Autodesk Fusion 360 part; units mm, degrees
note: some values were not read from the file. Set by a fixed rule: which sketch regions a step uses.
(part 3 of 7)
  spline S11 degree 5 poles (5.9883, 0.3741) (5.9868, 0.3751) (5.9838, 0.377) (5.9792, 0.3799) (5.9731, 0.3838) (5.9655, 0.3886) (5.9579, 0.3934) (5.9503, 0.3981) (5.9427, 0.4028) (5.9352, 0.4075) (5.9276, 0.4121) (5.92, 0.4167) (5.9125, 0.4213) (5.905, 0.4259) (5.8974, 0.4304) (5.8899, 0.4349) (5.8824, 0.4393) (5.8749, 0.4437) (5.8674, 0.4481) (5.8599, 0.4525) (5.8524, 0.4568) (5.845, 0.4611) (5.8375, 0.4654) (5.8301, 0.4696) (5.8226, 0.4738) (5.8152, 0.478) (5.8078, 0.4821) (5.8004, 0.4862) (5.793, 0.4903) (5.7856, 0.4943) (5.7782, 0.4984) (5.7709, 0.5023) (5.7635, 0.5063) (5.7562, 0.5102) (5.7489, 0.5141) (5.7416, 0.518) (5.7343, 0.5218) (5.727, 0.5256) (5.7197, 0.5293) (5.7124, 0.5331) (5.7052, 0.5368) (5.6979, 0.5405) (5.6907, 0.5441) (5.6835, 0.5477) (5.6763, 0.5513) (5.6691, 0.5548) (5.662, 0.5584) (5.6548, 0.5618) (5.6477, 0.5653) (5.6405, 0.5687) (5.6334, 0.5721) (5.6263, 0.5755) (5.6192, 0.5788) (5.6122, 0.5821) (5.6051, 0.5854) (5.5981, 0.5887) (5.5911, 0.5919) (5.584, 0.5951) (5.5771, 0.5982) (5.5701, 0.6013) (5.5631, 0.6044) (5.5562, 0.6075) (5.5492, 0.6105) (5.5423, 0.6136) (5.5354, 0.6165) (5.5286, 0.6195) (5.5217, 0.6224) (5.5149, 0.6253) (5.508, 0.6281) (5.5012, 0.631) (5.4945, 0.6338) (5.4877, 0.6366) (5.4809, 0.6393) (5.4742, 0.642) (5.4675, 0.6447) (5.4608, 0.6473) (5.4541, 0.65) (5.4475, 0.6526) (5.4408, 0.6551) (5.4342, 0.6577) (5.4276, 0.6602) (5.421, 0.6627) (5.4145, 0.6651) (5.4079, 0.6676) (5.4014, 0.67) (5.3949, 0.6723) (5.3884, 0.6747) (5.382, 0.677) (5.3756, 0.6793) (5.3691, 0.6815) (5.3628, 0.6838) (5.3564, 0.686) (5.35, 0.6882) (5.3437, 0.6903) (5.3374, 0.6924) (5.3311, 0.6945) (5.3249, 0.6966) (5.3186, 0.6986) (5.3124, 0.7006) (5.3063, 0.7026) (5.3001, 0.7046) (5.294, 0.7065) (5.2878, 0.7084) (5.2817, 0.7103) (5.2757, 0.7122) (5.2696, 0.714) (5.2636, 0.7158) (5.2576, 0.7176) (5.2517, 0.7193) (5.2457, 0.721) (5.2398, 0.7227) (5.2339, 0.7244) (5.2281, 0.726) (5.2222, 0.7277) (5.2164, 0.7293) (5.2106, 0.7308) (5.2049, 0.7324) (5.1991, 0.7339) (5.1934, 0.7354) (5.1878, 0.7368) (5.1821, 0.7383) (5.1765, 0.7397) (5.1709, 0.7411) (5.1653, 0.7425) (5.1598, 0.7438) (5.1543, 0.7451) (5.1488, 0.7464) (5.1434, 0.7477) (5.1379, 0.749) (5.1326, 0.7502) (5.1272, 0.7514) (5.1219, 0.7526) (5.1166, 0.7537) (5.1113, 0.7549) (5.1061, 0.756) (5.1009, 0.7571) (5.0957, 0.7581) (5.0905, 0.7592) (5.0854, 0.7602) (5.0803, 0.7612) (5.0753, 0.7622) (5.0703, 0.7631) (5.0653, 0.7641) (5.0604, 0.765) (5.0554, 0.7659) (5.0506, 0.7667) (5.0457, 0.7676) (5.0409, 0.7684) (5.0361, 0.7692) (5.0314, 0.77) (5.0266, 0.7708) (5.022, 0.7715) (5.0173, 0.7722) (5.0127, 0.7729) (5.0081, 0.7736) (5.0036, 0.7743) (4.9991, 0.7749) (4.9946, 0.7755) (4.9902, 0.7762) (4.9858, 0.7767) (4.9815, 0.7773) (4.9771, 0.7779) (4.9729, 0.7784) (4.9686, 0.7789) (4.9644, 0.7794) (4.9602, 0.7799) (4.9561, 0.7803) (4.952, 0.7808) (4.948, 0.7812) (4.944, 0.7816) (4.94, 0.782) (4.9361, 0.7824) (4.9322, 0.7828) (4.9283, 0.7831) (4.9245, 0.7834) (4.9207, 0.7838) (4.917, 0.784) (4.9133, 0.7843) (4.9097, 0.7846) (4.9061, 0.7849) (4.9025, 0.7851) (4.899, 0.7853) (4.8955, 0.7855) (4.8921, 0.7857) (4.8887, 0.7859) (4.8853, 0.7861) (4.882, 0.7862) (4.8788, 0.7864) (4.8756, 0.7865) (4.8724, 0.7866) (4.8693, 0.7867) (4.8662, 0.7868) (4.8632, 0.7869) (4.8602, 0.787) (4.8572, 0.7871) (4.8543, 0.7871) (4.8515, 0.7872) (4.8487, 0.7872) (4.846, 0.7872) (4.8433, 0.7872) (4.8406, 0.7872) (4.838, 0.7872) (4.8354, 0.7872) (4.8329, 0.7872) (4.8305, 0.7872) (4.8281, 0.7871) (4.8257, 0.7871) (4.8234, 0.787) (4.8211, 0.787) (4.8189, 0.7869) (4.8168, 0.7868) (4.8147, 0.7868) (4.8126, 0.7867) (4.8106, 0.7866) (4.8087, 0.7865) (4.8068, 0.7864) (4.805, 0.7863) (4.8032, 0.7862) (4.8015, 0.7861) (4.7998, 0.786) (4.7982, 0.7859) (4.7966, 0.7858) (4.7951, 0.7857) (4.7937, 0.7856) (4.7923, 0.7854) (4.7909, 0.7853) (4.7896, 0.7852) (4.7884, 0.7851) (4.7873, 0.785) (4.7862, 0.7849) (4.7851, 0.7848) (4.7841, 0.7847) (4.7832, 0.7846) (4.7824, 0.7845) (4.7816, 0.7844) (4.7808, 0.7843) (4.7801, 0.7842) (4.7795, 0.7841) (4.779, 0.7841) (4.7785, 0.784) (4.778, 0.7839) (4.7778, 0.7839) (4.7776, 0.7839) (4.7775, 0.7838) (4.7774, 0.7838) knots -1 -1 -1 -1 -1 -1 -0.99583333 -0.99166667 -0.9875 -0.98333333 -0.97916667 -0.975 -0.97083333 -0.96666667 -0.9625 -0.95833333 -0.95416667 -0.95 -0.94583333 -0.94166667 -0.9375 -0.93333333 -0.92916667 -0.925 -0.92083333 -0.91666667 -0.9125 -0.90833333 -0.90416667 -0.9 -0.89583333 -0.89166667 -0.8875 -0.88333333 -0.87916667 -0.875 -0.87083333 -0.86666667 -0.8625 -0.85833333 -0.85416667 -0.85 -0.84583333 -0.84166667 -0.8375 -0.83333333 -0.82916667 -0.825 -0.82083333 -0.81666667 -0.8125 -0.80833333 -0.80416667 -0.8 -0.79583333 -0.79166667 -0.7875 -0.78333333 -0.77916667 -0.775 -0.77083333 -0.76666667 -0.7625 -0.75833333 -0.75416667 -0.75 -0.74583333 -0.74166667 -0.7375 -0.73333333 -0.72916667 -0.725 -0.72083333 -0.71666667 -0.7125 -0.70833333 -0.70416667 -0.7 -0.69583333 -0.69166667 -0.6875 -0.68333333 -0.67916667 -0.675 -0.67083333 -0.66666667 -0.6625 -0.65833333 -0.65416667 -0.65 -0.64583333 -0.64166667 -0.6375 -0.63333333 -0.62916667 -0.625 -0.62083333 -0.61666667 -0.6125 -0.60833333 -0.60416667 -0.6 -0.59583333 -0.59166667 -0.5875 -0.58333333 -0.57916667 -0.575 -0.57083333 -0.56666667 -0.5625 -0.55833333 -0.55416667 -0.55 -0.54583333 -0.54166667 -0.5375 -0.53333333 -0.52916667 -0.525 -0.52083333 -0.51666667 -0.5125 -0.50833333 -0.50416667 -0.5 -0.49583333 -0.49166667 -0.4875 -0.48333333 -0.47916667 -0.475 -0.47083333 -0.46666667 -0.4625 -0.45833333 -0.45416667 -0.45 -0.44583333 -0.44166667 -0.4375 -0.43333333 -0.42916667 -0.425 -0.42083333 -0.41666667 -0.4125 -0.40833333 -0.40416667 -0.4 -0.39583333 -0.39166667 -0.3875 -0.38333333 -0.37916667 -0.375 -0.37083333 -0.36666667 -0.3625 -0.35833333 -0.35416667 -0.35 -0.34583333 -0.34166667 -0.3375 -0.33333333 -0.32916667 -0.325 -0.32083333 -0.31666667 -0.3125 -0.30833333 -0.30416667 -0.3 -0.29583333 -0.29166667 -0.2875 -0.28333333 -0.27916667 -0.275 -0.27083333 -0.26666667 -0.2625 -0.25833333 -0.25416667 -0.25 -0.24583333 -0.24166667 -0.2375 -0.23333333 -0.22916667 -0.225 -0.22083333 -0.21666667 -0.2125 -0.20833333 -0.20416667 -0.2 -0.19583333 -0.19166667 -0.1875 -0.18333333 -0.17916667 -0.175 -0.17083333 -0.16666667 -0.1625 -0.15833333 -0.15416667 -0.15 -0.14583333 -0.14166667 -0.1375 -0.13333333 -0.12916667 -0.125 -0.12083333 -0.11666667 -0.1125 -0.10833333 -0.10416667 -0.1 -0.09583333 -0.09166667 -0.0875 -0.08333333 -0.07916667 -0.075 -0.07083333 -0.06666667 -0.0625 -0.05833333 -0.05416667 -0.05 -0.04583333 -0.04166667 -0.0375 -0.03333333 -0.02916667 -0.025 -0.02083333 -0.01666667 -0.0125 -0.00833333 -0.00416667 0 0 0 0 0 0
  line L22 (4.7774, 0.7838) -> (4.7769, 0.7838)
  line L23 (4.7769, 0.7838) -> (3.7005, 0.6072)
  arc A12 (3.7005, 0.6072) -> (3.3507, 1.6839) centre (0, 0) ccw
  line L24 (3.3507, 1.6839) -> (4.3252, 2.1737)
  line L25 (4.3252, 2.1737) -> (4.3257, 2.1739)
  spline S12 degree 5 poles (4.3257, 2.1739) (4.3258, 2.174) (4.3259, 2.174) (4.326, 2.1741) (4.3263, 2.1742) (4.3267, 2.1745) (4.3271, 2.1747) (4.3276, 2.175) (4.3282, 2.1753) (4.3288, 2.1756) (4.3294, 2.1759) (4.3301, 2.1763) (4.3309, 2.1768) (4.3317, 2.1772) (4.3325, 2.1777) (4.3334, 2.1782) (4.3344, 2.1788) (4.3354, 2.1794) (4.3364, 2.18) (4.3375, 2.1807) (4.3387, 2.1814) (4.3399, 2.1821) (4.3411, 2.1829) (4.3424, 2.1837) (4.3437, 2.1845) (4.3451, 2.1854) (4.3465, 2.1863) (4.348, 2.1872) (4.3495, 2.1881) (4.351, 2.1891) (4.3526, 2.1902) (4.3542, 2.1913) (4.3559, 2.1924) (4.3576, 2.1935) (4.3593, 2.1947) (4.3611, 2.1959) (4.363, 2.1971) (4.3648, 2.1984) (4.3667, 2.1997) (4.3686, 2.2011) (4.3706, 2.2025) (4.3726, 2.2039) (4.3747, 2.2053) (4.3767, 2.2068) (4.3788, 2.2084) (4.381, 2.2099) (4.3832, 2.2115) (4.3854, 2.2132) (4.3876, 2.2148) (4.3899, 2.2165) (4.3922, 2.2183) (4.3946, 2.22) (4.3969, 2.2219) (4.3993, 2.2237) (4.4018, 2.2256) (4.4042, 2.2275) (4.4067, 2.2295) (4.4092, 2.2315) (4.4118, 2.2335) (4.4144, 2.2356) (4.417, 2.2377) (4.4196, 2.2398) (4.4223, 2.242) (4.425, 2.2442) (4.4277, 2.2465) (4.4304, 2.2488) (4.4332, 2.2511) (4.436, 2.2534) (4.4388, 2.2558) (4.4416, 2.2583) (4.4445, 2.2607) (4.4474, 2.2632) (4.4503, 2.2658) (4.4532, 2.2684) (4.4562, 2.271) (4.4592, 2.2736) (4.4622, 2.2763) (4.4652, 2.279) (4.4683, 2.2818) (4.4713, 2.2846) (4.4744, 2.2874) (4.4775, 2.2903) (4.4807, 2.2932) (4.4838, 2.2962) (4.487, 2.2992) (4.4902, 2.3022) (4.4934, 2.3052) (4.4966, 2.3083) (4.4998, 2.3115) (4.5031, 2.3146) (4.5064, 2.3178) (4.5097, 2.3211) (4.513, 2.3244) (4.5163, 2.3277) (4.5197, 2.331) (4.523, 2.3344) (4.5264, 2.3378) (4.5298, 2.3413) (4.5332, 2.3448) (4.5367, 2.3483) (4.5401, 2.3519) (4.5435, 2.3555) (4.547, 2.3592) (4.5505, 2.3629) (4.554, 2.3666) (4.5575, 2.3703) (4.561, 2.3741) (4.5646, 2.378) (4.5681, 2.3818) (4.5717, 2.3857) (4.5752, 2.3897) (4.5788, 2.3937) (4.5824, 2.3977) (4.586, 2.4017) (4.5896, 2.4058) (4.5933, 2.4099) (4.5969, 2.4141) (4.6006, 2.4183) (4.6042, 2.4225) (4.6079, 2.4268) (4.6116, 2.4311) (4.6153, 2.4354) (4.619, 2.4398) (4.6227, 2.4442) (4.6264, 2.4487) (4.6301, 2.4532) (4.6338, 2.4577) (4.6376, 2.4623) (4.6413, 2.4668) (4.645, 2.4715) (4.6488, 2.4761) (4.6526, 2.4809) (4.6563, 2.4856) (4.6601, 2.4904) (4.6639, 2.4952) (4.6677, 2.5) (4.6715, 2.5049) (4.6753, 2.5098) (4.6791, 2.5148) (4.6829, 2.5198) (4.6867, 2.5248) (4.6905, 2.5299) (4.6944, 2.535) (4.6982, 2.5401) (4.702, 2.5453) (4.7058, 2.5505) (4.7097, 2.5557) (4.7135, 2.561) (4.7174, 2.5663) (4.7212, 2.5717) (4.7251, 2.5771) (4.7289, 2.5825) (4.7328, 2.5879) (4.7366, 2.5934) (4.7405, 2.599) (4.7443, 2.6045) (4.7482, 2.6101) (4.7521, 2.6158) (4.7559, 2.6214) (4.7598, 2.6271) (4.7636, 2.6329) (4.7675, 2.6386) (4.7714, 2.6444) (4.7752, 2.6503) (4.7791, 2.6562) (4.7829, 2.6621) (4.7868, 2.668) (4.7907, 2.674) (4.7945, 2.68) (4.7984, 2.6861) (4.8022, 2.6921) (4.8061, 2.6983) (4.8099, 2.7044) (4.8138, 2.7106) (4.8176, 2.7168) (4.8215, 2.7231) (4.8253, 2.7294) (4.8292, 2.7357) (4.833, 2.7421) (4.8368, 2.7484) (4.8407, 2.7549) (4.8445, 2.7613) (4.8483, 2.7678) (4.8521, 2.7744) (4.8559, 2.7809) (4.8597, 2.7875) (4.8636, 2.7941) (4.8674, 2.8008) (4.8712, 2.8075) (4.8749, 2.8142) (4.8787, 2.821) (4.8825, 2.8278) (4.8863, 2.8346) (4.8901, 2.8415) (4.8938, 2.8484) (4.8976, 2.8553) (4.9013, 2.8623) (4.9051, 2.8693) (4.9088, 2.8763) (4.9125, 2.8834) (4.9163, 2.8905) (4.92, 2.8976) (4.9237, 2.9047) (4.9274, 2.9119) (4.9311, 2.9192) (4.9348, 2.9264) (4.9385, 2.9337) (4.9421, 2.941) (4.9458, 2.9484) (4.9495, 2.9558) (4.9531, 2.9632) (4.9568, 2.9706) (4.9604, 2.9781) (4.964, 2.9856) (4.9676, 2.9932) (4.9712, 3.0008) (4.9748, 3.0084) (4.9784, 3.016) (4.982, 3.0237) (4.9855, 3.0314) (4.9891, 3.0391) (4.9927, 3.0469) (4.9962, 3.0547) (4.9997, 3.0625) (5.0032, 3.0704) (5.0067, 3.0783) (5.0102, 3.0862) (5.0137, 3.0942) (5.0172, 3.1022) (5.0206, 3.1102) (5.0241, 3.1182) (5.0275, 3.1263) (5.031, 3.1344) (5.0344, 3.1426) (5.0378, 3.1507) (5.0412, 3.1589) (5.0445, 3.1672) (5.0479, 3.1754) (5.0513, 3.1837) (5.0546, 3.192) (5.0579, 3.2004) (5.0606, 3.2071) (5.0626, 3.2121) (5.0639, 3.2155) (5.0645, 3.2172) knots 0 0 0 0 0 0 0.00416667 0.00833333 0.0125 0.01666667 0.02083333 0.025 0.02916667 0.03333333 0.0375 0.04166667 0.04583333 0.05 0.05416667 0.05833333 0.0625 0.06666667 0.07083333 0.075 0.07916667 0.08333333 0.0875 0.09166667 0.09583333 0.1 0.10416667 0.10833333 0.1125 0.11666667 0.12083333 0.125 0.12916667 0.13333333 0.1375 0.14166667 0.14583333 0.15 0.15416667 0.15833333 0.1625 0.16666667 0.17083333 0.175 0.17916667 0.18333333 0.1875 0.19166667 0.19583333 0.2 0.20416667 0.20833333 0.2125 0.21666667 0.22083333 0.225 0.22916667 0.23333333 0.2375 0.24166667 0.24583333 0.25 0.25416667 0.25833333 0.2625 0.26666667 0.27083333 0.275 0.27916667 0.28333333 0.2875 0.29166667 0.29583333 0.3 0.30416667 0.30833333 0.3125 0.31666667 0.32083333 0.325 0.32916667 0.33333333 0.3375 0.34166667 0.34583333 0.35 0.35416667 0.35833333 0.3625 0.36666667 0.37083333 0.375 0.37916667 0.38333333 0.3875 0.39166667 0.39583333 0.4 0.40416667 0.40833333 0.4125 0.41666667 0.42083333 0.425 0.42916667 0.43333333 0.4375 0.44166667 0.44583333 0.45 0.45416667 0.45833333 0.4625 0.46666667 0.47083333 0.475 0.47916667 0.48333333 0.4875 0.49166667 0.49583333 0.5 0.50416667 0.50833333 0.5125 0.51666667 0.52083333 0.525 0.52916667 0.53333333 0.5375 0.54166667 0.54583333 0.55 0.55416667 0.55833333 0.5625 0.56666667 0.57083333 0.575 0.57916667 0.58333333 0.5875 0.59166667 0.59583333 0.6 0.60416667 0.60833333 0.6125 0.61666667 0.62083333 0.625 0.62916667 0.63333333 0.6375 0.64166667 0.64583333 0.65 0.65416667 0.65833333 0.6625 0.66666667 0.67083333 0.675 0.67916667 0.68333333 0.6875 0.69166667 0.69583333 0.7 0.70416667 0.70833333 0.7125 0.71666667 0.72083333 0.725 0.72916667 0.73333333 0.7375 0.74166667 0.74583333 0.75 0.75416667 0.75833333 0.7625 0.76666667 0.77083333 0.775 0.77916667 0.78333333 0.7875 0.79166667 0.79583333 0.8 0.80416667 0.80833333 0.8125 0.81666667 0.82083333 0.825 0.82916667 0.83333333 0.8375 0.84166667 0.84583333 0.85 0.85416667 0.85833333 0.8625 0.86666667 0.87083333 0.875 0.87916667 0.88333333 0.8875 0.89166667 0.89583333 0.9 0.90416667 0.90833333 0.9125 0.91666667 0.92083333 0.925 0.92916667 0.93333333 0.9375 0.94166667 0.94583333 0.95 0.95416667 0.95833333 0.9625 0.96666667 0.97083333 0.975 0.97916667 0.98333333 0.9875 0.99166667 0.99583333 1 1 1 1 1 1
  arc A13 (5.0645, 3.2172) -> (4.6248, 3.8225) centre (0, 0) ccw
  spline S13 degree 5 poles (4.6248, 3.8225) (4.623, 3.8224) (4.6194, 3.8222) (4.6139, 3.8218) (4.6067, 3.8214) (4.5978, 3.8208) (4.5888, 3.8202) (4.5799, 3.8196) (4.571, 3.8189) (4.5621, 3.8183) (4.5533, 3.8176) (4.5445, 3.8169) (4.5357, 3.8161) (4.5269, 3.8154) (4.5181, 3.8146) (4.5094, 3.8138) (4.5007, 3.813) (4.4921, 3.8122) (4.4834, 3.8113) (4.4748, 3.8104) (4.4662, 3.8095) (4.4576, 3.8086) (4.4491, 3.8077) (4.4406, 3.8067) (4.4321, 3.8058) (4.4236, 3.8048) (4.4152, 3.8038) (4.4068, 3.8027) (4.3984, 3.8017) (4.3901, 3.8006) (4.3818, 3.7995) (4.3735, 3.7984) (4.3652, 3.7973) (4.357, 3.7962) (4.3488, 3.795) (4.3406, 3.7938) (4.3324, 3.7926) (4.3243, 3.7914) (4.3162, 3.7902) (4.3081, 3.789) (4.3001, 3.7877) (4.2921, 3.7864) (4.2841, 3.7851) (4.2761, 3.7838) (4.2682, 3.7825) (4.2603, 3.7811) (4.2524, 3.7797) (4.2446, 3.7783) (4.2368, 3.7769) (4.229, 3.7755) (4.2212, 3.7741) (4.2135, 3.7727) (4.2058, 3.7712) (4.1982, 3.7697) (4.1905, 3.7682) (4.1829, 3.7667) (4.1754, 3.7652) (4.1678, 3.7636) (4.1603, 3.7621) (4.1528, 3.7605) (4.1454, 3.7589) (4.138, 3.7573) (4.1306, 3.7557) (4.1232, 3.7541) (4.1159, 3.7524) (4.1086, 3.7508) (4.1013, 3.7491) (4.0941, 3.7474) (4.0869, 3.7457) (4.0797, 3.744) (4.0726, 3.7423) (4.0655, 3.7406) (4.0584, 3.7388) (4.0514, 3.7371) (4.0444, 3.7353) (4.0374, 3.7335) (4.0304, 3.7317) (4.0235, 3.7299) (4.0166, 3.7281) (4.0098, 3.7262) (4.003, 3.7244) (3.9962, 3.7225) (3.9894, 3.7207) (3.9827, 3.7188) (3.976, 3.7169) (3.9694, 3.715) (3.9628, 3.7131) (3.9562, 3.7112) (3.9496, 3.7092) (3.9431, 3.7073) (3.9366, 3.7053) (3.9302, 3.7034) (3.9238, 3.7014) (3.9174, 3.6994) (3.9111, 3.6974) (3.9048, 3.6954) (3.8985, 3.6934) (3.8922, 3.6914) (3.886, 3.6894) (3.8799, 3.6874) (3.8737, 3.6853) (3.8676, 3.6833) (3.8615, 3.6812) (3.8555, 3.6792) (3.8495, 3.6771) (3.8436, 3.675) (3.8376, 3.673) (3.8317, 3.6709) (3.8259, 3.6688) (3.8201, 3.6667) (3.8143, 3.6646) (3.8085, 3.6625) (3.8028, 3.6604) (3.7972, 3.6582) (3.7915, 3.6561) (3.7859, 3.654) (3.7803, 3.6518) (3.7748, 3.6497) (3.7693, 3.6476) (3.7639, 3.6454) (3.7585, 3.6433) (3.7531, 3.6411) (3.7477, 3.6389) (3.7424, 3.6368) (3.7372, 3.6346) (3.7319, 3.6324) (3.7267, 3.6303) (3.7216, 3.6281) (3.7165, 3.6259) (3.7114, 3.6238) (3.7063, 3.6216) (3.7013, 3.6194) (3.6964, 3.6172) (3.6914, 3.615) (3.6865, 3.6129) (3.6817, 3.6107) (3.6769, 3.6085) (3.6721, 3.6063) (3.6674, 3.6041) (3.6627, 3.602) (3.658, 3.5998) (3.6534, 3.5976) (3.6488, 3.5954) (3.6443, 3.5933) (3.6398, 3.5911) (3.6353, 3.5889) (3.6309, 3.5868) (3.6265, 3.5846) (3.6222, 3.5824) (3.6179, 3.5803) (3.6136, 3.5781) (3.6094, 3.576) (3.6052, 3.5738) (3.6011, 3.5717) (3.5969, 3.5696) (3.5929, 3.5674) (3.5889, 3.5653) (3.5849, 3.5632) (3.5809, 3.5611) (3.577, 3.559) (3.5732, 3.5569) (3.5694, 3.5548) (3.5656, 3.5527) (3.5619, 3.5506) (3.5582, 3.5486) (3.5545, 3.5465) (3.5509, 3.5444) (3.5473, 3.5424) (3.5438, 3.5404) (3.5403, 3.5383) (3.5369, 3.5363) (3.5335, 3.5343) (3.5301, 3.5323) (3.5268, 3.5303) (3.5235, 3.5284) (3.5203, 3.5264) (3.5171, 3.5244) (3.5139, 3.5225) (3.5108, 3.5206) (3.5078, 3.5187) (3.5047, 3.5168) (3.5018, 3.5149) (3.4988, 3.513) (3.4959, 3.5112) (3.4931, 3.5093) (3.4903, 3.5075) (3.4875, 3.5057) (3.4848, 3.5039) (3.4821, 3.5021) (3.4795, 3.5003) (3.4769, 3.4986) (3.4743, 3.4968) (3.4718, 3.4951) (3.4694, 3.4934) (3.467, 3.4918) (3.4646, 3.4901) (3.4623, 3.4885) (3.46, 3.4868) (3.4577, 3.4852) (3.4556, 3.4837) (3.4534, 3.4821) (3.4513, 3.4806) (3.4492, 3.4791) (3.4472, 3.4776) (3.4453, 3.4761) (3.4433, 3.4747) (3.4414, 3.4732) (3.4396, 3.4718) (3.4378, 3.4705) (3.4361, 3.4691) (3.4344, 3.4678) (3.4327, 3.4665) (3.4311, 3.4652) (3.4295, 3.464) (3.428, 3.4628) (3.4265, 3.4616) (3.4251, 3.4604) (3.4237, 3.4593) (3.4224, 3.4582) (3.4211, 3.4571) (3.4199, 3.4561) (3.4187, 3.4551) (3.4175, 3.4541) (3.4164, 3.4532) (3.4153, 3.4523) (3.4143, 3.4514) (3.4134, 3.4505) (3.4124, 3.4497) (3.4116, 3.449) (3.4107, 3.4482) (3.41, 3.4475) (3.4092, 3.4469) (3.4085, 3.4462) (3.4079, 3.4457) (3.4073, 3.4451) (3.4068, 3.4446) (3.4063, 3.4441) (3.4058, 3.4437) (3.4054, 3.4433) (3.405, 3.443) (3.4047, 3.4427) (3.4045, 3.4425) (3.4044, 3.4423) (3.4043, 3.4423) (3.4043, 3.4422) knots -1 -1 -1 -1 -1 -1 -0.99583333 -0.99166667 -0.9875 -0.98333333 -0.97916667 -0.975 -0.97083333 -0.96666667 -0.9625 -0.95833333 -0.95416667 -0.95 -0.94583333 -0.94166667 -0.9375 -0.93333333 -0.92916667 -0.925 -0.92083333 -0.91666667 -0.9125 -0.90833333 -0.90416667 -0.9 -0.89583333 -0.89166667 -0.8875 -0.88333333 -0.87916667 -0.875 -0.87083333 -0.86666667 -0.8625 -0.85833333 -0.85416667 -0.85 -0.84583333 -0.84166667 -0.8375 -0.83333333 -0.82916667 -0.825 -0.82083333 -0.81666667 -0.8125 -0.80833333 -0.80416667 -0.8 -0.79583333 -0.79166667 -0.7875 -0.78333333 -0.77916667 -0.775 -0.77083333 -0.76666667 -0.7625 -0.75833333 -0.75416667 -0.75 -0.74583333 -0.74166667 -0.7375 -0.73333333 -0.72916667 -0.725 -0.72083333 -0.71666667 -0.7125 -0.70833333 -0.70416667 -0.7 -0.69583333 -0.69166667 -0.6875 -0.68333333 -0.67916667 -0.675 -0.67083333 -0.66666667 -0.6625 -0.65833333 -0.65416667 -0.65 -0.64583333 -0.64166667 -0.6375 -0.63333333 -0.62916667 -0.625 -0.62083333 -0.61666667 -0.6125 -0.60833333 -0.60416667 -0.6 -0.59583333 -0.59166667 -0.5875 -0.58333333 -0.57916667 -0.575 -0.57083333 -0.56666667 -0.5625 -0.55833333 -0.55416667 -0.55 -0.54583333 -0.54166667 -0.5375 -0.53333333 -0.52916667 -0.525 -0.52083333 -0.51666667 -0.5125 -0.50833333 -0.50416667 -0.5 -0.49583333 -0.49166667 -0.4875 -0.48333333 -0.47916667 -0.475 -0.47083333 -0.46666667 -0.4625 -0.45833333 -0.45416667 -0.45 -0.44583333 -0.44166667 -0.4375 -0.43333333 -0.42916667 -0.425 -0.42083333 -0.41666667 -0.4125 -0.40833333 -0.40416667 -0.4 -0.39583333 -0.39166667 -0.3875 -0.38333333 -0.37916667 -0.375 -0.37083333 -0.36666667 -0.3625 -0.35833333 -0.35416667 -0.35 -0.34583333 -0.34166667 -0.3375 -0.33333333 -0.32916667 -0.325 -0.32083333 -0.31666667 -0.3125 -0.30833333 -0.30416667 -0.3 -0.29583333 -0.29166667 -0.2875 -0.28333333 -0.27916667 -0.275 -0.27083333 -0.26666667 -0.2625 -0.25833333 -0.25416667 -0.25 -0.24583333 -0.24166667 -0.2375 -0.23333333 -0.22916667 -0.225 -0.22083333 -0.21666667 -0.2125 -0.20833333 -0.20416667 -0.2 -0.19583333 -0.19166667 -0.1875 -0.18333333 -0.17916667 -0.175 -0.17083333 -0.16666667 -0.1625 -0.15833333 -0.15416667 -0.15 -0.14583333 -0.14166667 -0.1375 -0.13333333 -0.12916667 -0.125 -0.12083333 -0.11666667 -0.1125 -0.10833333 -0.10416667 -0.1 -0.09583333 -0.09166667 -0.0875 -0.08333333 -0.07916667 -0.075 -0.07083333 -0.06666667 -0.0625 -0.05833333 -0.05416667 -0.05 -0.04583333 -0.04166667 -0.0375 -0.03333333 -0.02916667 -0.025 -0.02083333 -0.01666667 -0.0125 -0.00833333 -0.00416667 0 0 0 0 0 0
  line L26 (3.4043, 3.4422) -> (3.4039, 3.4418)
  line L27 (3.4039, 3.4418) -> (2.6369, 2.6663)
  arc A14 (2.6369, 2.6663) -> (1.721, 3.3318) centre (0, 0) ccw
  line L28 (1.721, 3.3318) -> (2.2215, 4.3009)
  line L29 (2.2215, 4.3009) -> (2.2218, 4.3014)
  spline S14 degree 5 poles (2.2218, 4.3014) (2.2218, 4.3014) (2.2218, 4.3015) (2.2219, 4.3017) (2.2221, 4.3019) (2.2223, 4.3023) (2.2225, 4.3028) (2.2227, 4.3033) (2.223, 4.3038) (2.2233, 4.3045) (2.2236, 4.3051) (2.2239, 4.3059) (2.2243, 4.3067) (2.2247, 4.3075) (2.2251, 4.3084) (2.2255, 4.3094) (2.2259, 4.3104) (2.2264, 4.3115) (2.2269, 4.3126) (2.2274, 4.3138) (2.2279, 4.315) (2.2284, 4.3163) (2.229, 4.3176) (2.2296, 4.319) (2.2301, 4.3205) (2.2307, 4.322) (2.2314, 4.3235) (2.232, 4.3251) (2.2326, 4.3268) (2.2333, 4.3285) (2.234, 4.3303) (2.2347, 4.3321) (2.2354, 4.334) (2.2361, 4.3359) (2.2368, 4.3379) (2.2375, 4.3399) (2.2383, 4.342) (2.239, 4.3441) (2.2398, 4.3463) (2.2405, 4.3485) (2.2413, 4.3508) (2.2421, 4.3531) (2.2429, 4.3555) (2.2437, 4.3579) (2.2445, 4.3604) (2.2453, 4.3629) (2.2462, 4.3655) (2.247, 4.3681) (2.2478, 4.3708) (2.2487, 4.3735) (2.2495, 4.3763) (2.2504, 4.3791) (2.2512, 4.382) (2.2521, 4.3849) (2.2529, 4.3878) (2.2538, 4.3908) (2.2547, 4.3939) (2.2555, 4.397) (2.2564, 4.4001) (2.2573, 4.4033) (2.2581, 4.4066) (2.259, 4.4098) (2.2599, 4.4132) (2.2608, 4.4165) (2.2616, 4.4199) (2.2625, 4.4234) (2.2634, 4.4269) (2.2642, 4.4305) (2.2651, 4.4341) (2.266, 4.4377) (2.2668, 4.4414) (2.2677, 4.4451) (2.2686, 4.4489) (2.2694, 4.4527) (2.2703, 4.4565) (2.2711, 4.4604) (2.272, 4.4644) (2.2728, 4.4684) (2.2737, 4.4724) (2.2745, 4.4765) (2.2753, 4.4806) (2.2762, 4.4847) (2.277, 4.4889) (2.2778, 4.4932) (2.2786, 4.4974) (2.2794, 4.5018) (2.2802, 4.5061) (2.281, 4.5105) (2.2818, 4.515) (2.2826, 4.5194) (2.2833, 4.524) (2.2841, 4.5285) (2.2849, 4.5331) (2.2856, 4.5378) (2.2863, 4.5424) (2.2871, 4.5472) (2.2878, 4.5519) (2.2885, 4.5567) (2.2892, 4.5616) (2.2899, 4.5664) (2.2906, 4.5713) (2.2913, 4.5763) (2.2919, 4.5813) (2.2926, 4.5863) (2.2932, 4.5914) (2.2938, 4.5965) (2.2945, 4.6016) (2.2951, 4.6068) (2.2957, 4.612) (2.2963, 4.6173) (2.2968, 4.6225) (2.2974, 4.6279) (2.2979, 4.6332) (2.2985, 4.6386) (2.299, 4.6441) (2.2995, 4.6495) (2.3, 4.655) (2.3005, 4.6606) (2.301, 4.6661) (2.3014, 4.6718) (2.3019, 4.6774) (2.3023, 4.6831) (2.3027, 4.6888) (2.3031, 4.6945) (2.3035, 4.7003) (2.3039, 4.7062) (2.3042, 4.712) (2.3046, 4.7179) (2.3049, 4.7238) (2.3052, 4.7298) (2.3055, 4.7357) (2.3058, 4.7418) (2.3061, 4.7478) (2.3063, 4.7539) (2.3065, 4.76) (2.3068, 4.7662) (2.307, 4.7724) (2.3071, 4.7786) (2.3073, 4.7848) (2.3074, 4.7911) (2.3076, 4.7974) (2.3077, 4.8037) (2.3078, 4.8101) (2.3079, 4.8165) (2.3079, 4.823) (2.308, 4.8294) (2.308, 4.8359) (2.308, 4.8424) (2.308, 4.849) (2.3079, 4.8556) (2.3079, 4.8622) (2.3078, 4.8689) (2.3077, 4.8755) (2.3076, 4.8822) (2.3075, 4.889) (2.3073, 4.8958) (2.3072, 4.9025) (2.307, 4.9094) (2.3068, 4.9162) (2.3066, 4.9231) (2.3063, 4.93) (2.306, 4.937) (2.3057, 4.9439) (2.3054, 4.9509) (2.3051, 4.9579) (2.3048, 4.965) (2.3044, 4.9721) (2.304, 4.9792) (2.3036, 4.9863) (2.3031, 4.9935) (2.3027, 5.0007) (2.3022, 5.0079) (2.3017, 5.0151) (2.3012, 5.0224) (2.3006, 5.0297) (2.3001, 5.037) (2.2995, 5.0444) (2.2989, 5.0517) (2.2982, 5.0591) (2.2976, 5.0666) (2.2969, 5.074) (2.2962, 5.0815) (2.2955, 5.089) (2.2947, 5.0965) (2.294, 5.1041) (2.2932, 5.1116) (2.2923, 5.1192) (2.2915, 5.1269) (2.2906, 5.1345) (2.2897, 5.1422) (2.2888, 5.1499) (2.2879, 5.1576) (2.2869, 5.1653) (2.286, 5.1731) (2.2849, 5.1809) (2.2839, 5.1887) (2.2829, 5.1966) (2.2818, 5.2044) (2.2807, 5.2123) (2.2795, 5.2202) (2.2784, 5.2281) (2.2772, 5.2361) (2.276, 5.2441) (2.2748, 5.2521) (2.2735, 5.2601) (2.2722, 5.2681) (2.2709, 5.2762) (2.2696, 5.2843) (2.2682, 5.2924) (2.2668, 5.3005) (2.2654, 5.3086) (2.264, 5.3168) (2.2625, 5.325) (2.2611, 5.3332) (2.2595, 5.3414) (2.258, 5.3497) (2.2564, 5.358) (2.2548, 5.3662) (2.2532, 5.3746) (2.2516, 5.3829) (2.2499, 5.3912) (2.2482, 5.3996) (2.2465, 5.408) (2.2447, 5.4164) (2.243, 5.4248) (2.2412, 5.4333) (2.2393, 5.4417) (2.2375, 5.4502) (2.2356, 5.4587) (2.2337, 5.4672) (2.2317, 5.4758) (2.2298, 5.4843) (2.2278, 5.4929) (2.2257, 5.5015) (2.2237, 5.5101) (2.2216, 5.5188) (2.2195, 5.5274) (2.2174, 5.5361) (2.2152, 5.5447) (2.213, 5.5534) (2.2108, 5.5622) (2.209, 5.5691) (2.2076, 5.5744) (2.2067, 5.5779) (2.2063, 5.5796) knots 0 0 0 0 0 0 0.00416667 0.00833333 0.0125 0.01666667 0.02083333 0.025 0.02916667 0.03333333 0.0375 0.04166667 0.04583333 0.05 0.05416667 0.05833333 0.0625 0.06666667 0.07083333 0.075 0.07916667 0.08333333 0.0875 0.09166667 0.09583333 0.1 0.10416667 0.10833333 0.1125 0.11666667 0.12083333 0.125 0.12916667 0.13333333 0.1375 0.14166667 0.14583333 0.15 0.15416667 0.15833333 0.1625 0.16666667 0.17083333 0.175 0.17916667 0.18333333 0.1875 0.19166667 0.19583333 0.2 0.20416667 0.20833333 0.2125 0.21666667 0.22083333 0.225 0.22916667 0.23333333 0.2375 0.24166667 0.24583333 0.25 0.25416667 0.25833333 0.2625 0.26666667 0.27083333 0.275 0.27916667 0.28333333 0.2875 0.29166667 0.29583333 0.3 0.30416667 0.30833333 0.3125 0.31666667 0.32083333 0.325 0.32916667 0.33333333 0.3375 0.34166667 0.34583333 0.35 0.35416667 0.35833333 0.3625 0.36666667 0.37083333 0.375 0.37916667 0.38333333 0.3875 0.39166667 0.39583333 0.4 0.40416667 0.40833333 0.4125 0.41666667 0.42083333 0.425 0.42916667 0.43333333 0.4375 0.44166667 0.44583333 0.45 0.45416667 0.45833333 0.4625 0.46666667 0.47083333 0.475 0.47916667 0.48333333 0.4875 0.49166667 0.49583333 0.5 0.50416667 0.50833333 0.5125 0.51666667 0.52083333 0.525 0.52916667 0.53333333 0.5375 0.54166667 0.54583333 0.55 0.55416667 0.55833333 0.5625 0.56666667 0.57083333 0.575 0.57916667 0.58333333 0.5875 0.59166667 0.59583333 0.6 0.60416667 0.60833333 0.6125 0.61666667 0.62083333 0.625 0.62916667 0.63333333 0.6375 0.64166667 0.64583333 0.65 0.65416667 0.65833333 0.6625 0.66666667 0.67083333 0.675 0.67916667 0.68333333 0.6875 0.69166667 0.69583333 0.7 0.70416667 0.70833333 0.7125 0.71666667 0.72083333 0.725 0.72916667 0.73333333 0.7375 0.74166667 0.74583333 0.75 0.75416667 0.75833333 0.7625 0.76666667 0.77083333 0.775 0.77916667 0.78333333 0.7875 0.79166667 0.79583333 0.8 0.80416667 0.80833333 0.8125 0.81666667 0.82083333 0.825 0.82916667 0.83333333 0.8375 0.84166667 0.84583333 0.85 0.85416667 0.85833333 0.8625 0.86666667 0.87083333 0.875 0.87916667 0.88333333 0.8875 0.89166667 0.89583333 0.9 0.90416667 0.90833333 0.9125 0.91666667 0.92083333 0.925 0.92916667 0.93333333 0.9375 0.94166667 0.94583333 0.95 0.95416667 0.95833333 0.9625 0.96666667 0.97083333 0.975 0.97916667 0.98333333 0.9875 0.99166667 0.99583333 1 1 1 1 1 1
  arc A15 (2.2063, 5.5796) -> (1.4947, 5.8108) centre (0, 0) ccw
  spline S15 degree 5 poles (1.4947, 5.8108) (1.4933, 5.8097) (1.4905, 5.8074) (1.4863, 5.8039) (1.4808, 5.7994) (1.4739, 5.7936) (1.467, 5.7879) (1.4601, 5.7821) (1.4533, 5.7764) (1.4465, 5.7706) (1.4398, 5.7648) (1.433, 5.7591) (1.4264, 5.7533) (1.4197, 5.7475) (1.4131, 5.7418) (1.4065, 5.736) (1.3999, 5.7302) (1.3934, 5.7245) (1.3869, 5.7187) (1.3805, 5.7129) (1.374, 5.7072) (1.3676, 5.7014) (1.3613, 5.6956) (1.355, 5.6898) (1.3487, 5.6841) (1.3424, 5.6783) (1.3362, 5.6725) (1.33, 5.6667) (1.3238, 5.661) (1.3177, 5.6552) (1.3116, 5.6494) (1.3055, 5.6437) (1.2995, 5.6379) (1.2935, 5.6321) (1.2876, 5.6264) (1.2816, 5.6206) (1.2757, 5.6148) (1.2699, 5.6091) (1.264, 5.6033) (1.2583, 5.5976) (1.2525, 5.5918) (1.2468, 5.5861) (1.2411, 5.5803) (1.2354, 5.5746) (1.2298, 5.5688) (1.2242, 5.5631) (1.2186, 5.5574) (1.2131, 5.5517) (1.2076, 5.5459) (1.2021, 5.5402) (1.1967, 5.5345) (1.1913, 5.5288) (1.1859, 5.5231) (1.1806, 5.5174) (1.1753, 5.5117) (1.1701, 5.506) (1.1648, 5.5003) (1.1596, 5.4946) (1.1545, 5.489) (1.1493, 5.4833) (1.1442, 5.4776) (1.1392, 5.472) (1.1342, 5.4663) (1.1292, 5.4607) (1.1242, 5.455) (1.1193, 5.4494) (1.1144, 5.4438) (1.1095, 5.4382) (1.1047, 5.4326) (1.0999, 5.427) (1.0951, 5.4214) (1.0904, 5.4158) (1.0857, 5.4102) (1.081, 5.4047) (1.0764, 5.3991) (1.0718, 5.3936) (1.0673, 5.388) (1.0627, 5.3825) (1.0582, 5.377) (1.0538, 5.3715) (1.0493, 5.366) (1.0449, 5.3605) (1.0406, 5.355) (1.0362, 5.3495) (1.032, 5.3441) (1.0277, 5.3386) (1.0235, 5.3332) (1.0193, 5.3278) (1.0151, 5.3224) (1.011, 5.317) (1.0069, 5.3116) (1.0028, 5.3062) (0.9988, 5.3008) (0.9948, 5.2955) (0.9908, 5.2902) (0.9869, 5.2848) (0.983, 5.2795) (0.9791, 5.2742) (0.9753, 5.2689) (0.9715, 5.2637) (0.9677, 5.2584) (0.964, 5.2532) (0.9603, 5.2479) (0.9566, 5.2427) (0.953, 5.2375) (0.9494, 5.2324) (0.9458, 5.2272) (0.9423, 5.222) (0.9388, 5.2169) (0.9353, 5.2118) (0.9318, 5.2067) (0.9284, 5.2016) (0.9251, 5.1965) (0.9217, 5.1915) (0.9184, 5.1864) (0.9151, 5.1814) (0.9119, 5.1764) (0.9087, 5.1715) (0.9055, 5.1665) (0.9023, 5.1615) (0.8992, 5.1566) (0.8961, 5.1517) (0.8931, 5.1468) (0.89, 5.142) (0.8871, 5.1371) (0.8841, 5.1323) (0.8812, 5.1275) (0.8783, 5.1227) (0.8754, 5.1179) (0.8726, 5.1132) (0.8698, 5.1084) (0.867, 5.1037) (0.8643, 5.0991) (0.8616, 5.0944) (0.8589, 5.0898) (0.8562, 5.0852) (0.8536, 5.0806) (0.851, 5.076) (0.8485, 5.0714) (0.846, 5.0669) (0.8435, 5.0624) (0.841, 5.0579) (0.8386, 5.0535) (0.8362, 5.0491) (0.8338, 5.0447) (0.8315, 5.0403) (0.8292, 5.0359) (0.8269, 5.0316) (0.8247, 5.0273) (0.8225, 5.023) (0.8203, 5.0188) (0.8181, 5.0146) (0.816, 5.0104) (0.8139, 5.0062) (0.8119, 5.0021) (0.8098, 4.998) (0.8078, 4.9939) (0.8058, 4.9898) (0.8039, 4.9858) (0.802, 4.9818) (0.8001, 4.9778) (0.7982, 4.9739) (0.7964, 4.97) (0.7946, 4.9661) (0.7928, 4.9623) (0.7911, 4.9585) (0.7894, 4.9547) (0.7877, 4.9509) (0.786, 4.9472) (0.7844, 4.9435) (0.7828, 4.9399) (0.7812, 4.9362) (0.7797, 4.9327) (0.7782, 4.9291) (0.7767, 4.9256) (0.7752, 4.9221) (0.7738, 4.9186) (0.7724, 4.9152) (0.771, 4.9118) (0.7696, 4.9085) (0.7683, 4.9052) (0.767, 4.9019) (0.7657, 4.8986) (0.7645, 4.8954) (0.7632, 4.8923) (0.762, 4.8891) (0.7609, 4.8861) (0.7597, 4.883) (0.7586, 4.88) (0.7575, 4.877) (0.7565, 4.8741) (0.7554, 4.8712) (0.7544, 4.8683) (0.7534, 4.8655) (0.7524, 4.8627) (0.7515, 4.86) (0.7506, 4.8573) (0.7497, 4.8546) (0.7488, 4.852) (0.748, 4.8495) (0.7471, 4.8469) (0.7463, 4.8445) (0.7456, 4.842) (0.7448, 4.8396) (0.7441, 4.8373) (0.7434, 4.835) (0.7427, 4.8327) (0.742, 4.8305) (0.7414, 4.8284) (0.7407, 4.8262) (0.7401, 4.8242) (0.7396, 4.8222) (0.739, 4.8202) (0.7385, 4.8183) (0.738, 4.8164) (0.7375, 4.8146) (0.737, 4.8128) (0.7365, 4.8111) (0.7361, 4.8094) (0.7357, 4.8078) (0.7353, 4.8062) (0.7349, 4.8047) (0.7345, 4.8032) (0.7342, 4.8018) (0.7339, 4.8004) (0.7336, 4.7991) (0.7333, 4.7979) (0.733, 4.7967) (0.7328, 4.7955) (0.7325, 4.7945) (0.7323, 4.7934) (0.7321, 4.7925) (0.7319, 4.7916) (0.7317, 4.7907) (0.7316, 4.7899) (0.7314, 4.7892) (0.7313, 4.7885) (0.7312, 4.7879) (0.7311, 4.7874) (0.731, 4.7869) (0.7309, 4.7864) (0.7309, 4.7862) (0.7309, 4.786) (0.7308, 4.7859) (0.7308, 4.7858) knots -1 -1 -1 -1 -1 -1 -0.99583333 -0.99166667 -0.9875 -0.98333333 -0.97916667 -0.975 -0.97083333 -0.96666667 -0.9625 -0.95833333 -0.95416667 -0.95 -0.94583333 -0.94166667 -0.9375 -0.93333333 -0.92916667 -0.925 -0.92083333 -0.91666667 -0.9125 -0.90833333 -0.90416667 -0.9 -0.89583333 -0.89166667 -0.8875 -0.88333333 -0.87916667 -0.875 -0.87083333 -0.86666667 -0.8625 -0.85833333 -0.85416667 -0.85 -0.84583333 -0.84166667 -0.8375 -0.83333333 -0.82916667 -0.825 -0.82083333 -0.81666667 -0.8125 -0.80833333 -0.80416667 -0.8 -0.79583333 -0.79166667 -0.7875 -0.78333333 -0.77916667 -0.775 -0.77083333 -0.76666667 -0.7625 -0.75833333 -0.75416667 -0.75 -0.74583333 -0.74166667 -0.7375 -0.73333333 -0.72916667 -0.725 -0.72083333 -0.71666667 -0.7125 -0.70833333 -0.70416667 -0.7 -0.69583333 -0.69166667 -0.6875 -0.68333333 -0.67916667 -0.675 -0.67083333 -0.66666667 -0.6625 -0.65833333 -0.65416667 -0.65 -0.64583333 -0.64166667 -0.6375 -0.63333333 -0.62916667 -0.625 -0.62083333 -0.61666667 -0.6125 -0.60833333 -0.60416667 -0.6 -0.59583333 -0.59166667 -0.5875 -0.58333333 -0.57916667 -0.575 -0.57083333 -0.56666667 -0.5625 -0.55833333 -0.55416667 -0.55 -0.54583333 -0.54166667 -0.5375 -0.53333333 -0.52916667 -0.525 -0.52083333 -0.51666667 -0.5125 -0.50833333 -0.50416667 -0.5 -0.49583333 -0.49166667 -0.4875 -0.48333333 -0.47916667 -0.475 -0.47083333 -0.46666667 -0.4625 -0.45833333 -0.45416667 -0.45 -0.44583333 -0.44166667 -0.4375 -0.43333333 -0.42916667 -0.425 -0.42083333 -0.41666667 -0.4125 -0.40833333 -0.40416667 -0.4 -0.39583333 -0.39166667 -0.3875 -0.38333333 -0.37916667 -0.375 -0.37083333 -0.36666667 -0.3625 -0.35833333 -0.35416667 -0.35 -0.34583333 -0.34166667 -0.3375 -0.33333333 -0.32916667 -0.325 -0.32083333 -0.31666667 -0.3125 -0.30833333 -0.30416667 -0.3 -0.29583333 -0.29166667 -0.2875 -0.28333333 -0.27916667 -0.275 -0.27083333 -0.26666667 -0.2625 -0.25833333 -0.25416667 -0.25 -0.24583333 -0.24166667 -0.2375 -0.23333333 -0.22916667 -0.225 -0.22083333 -0.21666667 -0.2125 -0.20833333 -0.20416667 -0.2 -0.19583333 -0.19166667 -0.1875 -0.18333333 -0.17916667 -0.175 -0.17083333 -0.16666667 -0.1625 -0.15833333 -0.15416667 -0.15 -0.14583333 -0.14166667 -0.1375 -0.13333333 -0.12916667 -0.125 -0.12083333 -0.11666667 -0.1125 -0.10833333 -0.10416667 -0.1 -0.09583333 -0.09166667 -0.0875 -0.08333333 -0.07916667 -0.075 -0.07083333 -0.06666667 -0.0625 -0.05833333 -0.05416667 -0.05 -0.04583333 -0.04166667 -0.0375 -0.03333333 -0.02916667 -0.025 -0.02083333 -0.01666667 -0.0125 -0.00833333 -0.00416667 0 0 0 0 0 0
  line L30 (0.7308, 4.7858) -> (0.7307, 4.7853)
  line L31 (0.7307, 4.7853) -> (0.5661, 3.707)
  arc A16 (0.5661, 3.707) -> (-0.5661, 3.707) centre (0, 0) ccw
  line L32 (-0.5661, 3.707) -> (-0.7307, 4.7853)
  line L33 (-0.7307, 4.7853) -> (-0.7308, 4.7858)
  spline S16 degree 5 poles (-0.7308, 4.7858) (-0.7308, 4.7859) (-0.7309, 4.786) (-0.7309, 4.7862) (-0.7309, 4.7864) (-0.731, 4.7869) (-0.7311, 4.7874) (-0.7312, 4.7879) (-0.7313, 4.7885) (-0.7314, 4.7892) (-0.7316, 4.7899) (-0.7317, 4.7907) (-0.7319, 4.7916) (-0.7321, 4.7925) (-0.7323, 4.7934) (-0.7325, 4.7945) (-0.7328, 4.7955) (-0.733, 4.7967) (-0.7333, 4.7979) (-0.7336, 4.7991) (-0.7339, 4.8004) (-0.7342, 4.8018) (-0.7345, 4.8032) (-0.7349, 4.8047) (-0.7353, 4.8062) (-0.7357, 4.8078) (-0.7361, 4.8094) (-0.7365, 4.8111) (-0.737, 4.8128) (-0.7375, 4.8146) (-0.738, 4.8164) (-0.7385, 4.8183) (-0.739, 4.8202) (-0.7396, 4.8222) (-0.7401, 4.8242) (-0.7407, 4.8262) (-0.7414, 4.8284) (-0.742, 4.8305) (-0.7427, 4.8327) (-0.7434, 4.835) (-0.7441, 4.8373) (-0.7448, 4.8396) (-0.7456, 4.842) (-0.7463, 4.8445) (-0.7471, 4.8469) (-0.748, 4.8495) (-0.7488, 4.852) (-0.7497, 4.8546) (-0.7506, 4.8573) (-0.7515, 4.86) (-0.7524, 4.8627) (-0.7534, 4.8655) (-0.7544, 4.8683) (-0.7554, 4.8712) (-0.7565, 4.8741) (-0.7575, 4.877) (-0.7586, 4.88) (-0.7597, 4.883) (-0.7609, 4.8861) (-0.762, 4.8891) (-0.7632, 4.8923) (-0.7645, 4.8954) (-0.7657, 4.8986) (-0.767, 4.9019) (-0.7683, 4.9052) (-0.7696, 4.9085) (-0.771, 4.9118) (-0.7724, 4.9152) (-0.7738, 4.9186) (-0.7752, 4.9221) (-0.7767, 4.9256) (-0.7782, 4.9291) (-0.7797, 4.9327) (-0.7812, 4.9362) (-0.7828, 4.9399) (-0.7844, 4.9435) (-0.786, 4.9472) (-0.7877, 4.9509) (-0.7894, 4.9547) (-0.7911, 4.9585) (-0.7928, 4.9623) (-0.7946, 4.9661) (-0.7964, 4.97) (-0.7982, 4.9739) (-0.8001, 4.9778) (-0.802, 4.9818) (-0.8039, 4.9858) (-0.8058, 4.9898) (-0.8078, 4.9939) (-0.8098, 4.998) (-0.8119, 5.0021) (-0.8139, 5.0062) (-0.816, 5.0104) (-0.8181, 5.0146) (-0.8203, 5.0188) (-0.8225, 5.023) (-0.8247, 5.0273) (-0.8269, 5.0316) (-0.8292, 5.0359) (-0.8315, 5.0403) (-0.8338, 5.0447) (-0.8362, 5.0491) (-0.8386, 5.0535) (-0.841, 5.0579) (-0.8435, 5.0624) (-0.846, 5.0669) (-0.8485, 5.0714) (-0.851, 5.076) (-0.8536, 5.0806) (-0.8562, 5.0852) (-0.8589, 5.0898) (-0.8616, 5.0944) (-0.8643, 5.0991) (-0.867, 5.1037) (-0.8698, 5.1084) (-0.8726, 5.1132) (-0.8754, 5.1179) (-0.8783, 5.1227) (-0.8812, 5.1275) (-0.8841, 5.1323) (-0.8871, 5.1371) (-0.89, 5.142) (-0.8931, 5.1468) (-0.8961, 5.1517) (-0.8992, 5.1566) (-0.9023, 5.1615) (-0.9055, 5.1665) (-0.9087, 5.1715) (-0.9119, 5.1764) (-0.9151, 5.1814) (-0.9184, 5.1864) (-0.9217, 5.1915) (-0.9251, 5.1965) (-0.9284, 5.2016) (-0.9318, 5.2067) (-0.9353, 5.2118) (-0.9388, 5.2169) (-0.9423, 5.222) (-0.9458, 5.2272) (-0.9494, 5.2324) (-0.953, 5.2375) (-0.9566, 5.2427) (-0.9603, 5.2479) (-0.964, 5.2532) (-0.9677, 5.2584) (-0.9715, 5.2637) (-0.9753, 5.2689) (-0.9791, 5.2742) (-0.983, 5.2795) (-0.9869, 5.2848) (-0.9908, 5.2902) (-0.9948, 5.2955) (-0.9988, 5.3008) (-1.0028, 5.3062) (-1.0069, 5.3116) (-1.011, 5.317) (-1.0151, 5.3224) (-1.0193, 5.3278) (-1.0235, 5.3332) (-1.0277, 5.3386) (-1.032, 5.3441) (-1.0362, 5.3495) (-1.0406, 5.355) (-1.0449, 5.3605) (-1.0493, 5.366) (-1.0538, 5.3715) (-1.0582, 5.377) (-1.0627, 5.3825) (-1.0673, 5.388) (-1.0718, 5.3936) (-1.0764, 5.3991) (-1.081, 5.4047) (-1.0857, 5.4102) (-1.0904, 5.4158) (-1.0951, 5.4214) (-1.0999, 5.427) (-1.1047, 5.4326) (-1.1095, 5.4382) (-1.1144, 5.4438) (-1.1193, 5.4494) (-1.1242, 5.455) (-1.1292, 5.4607) (-1.1342, 5.4663) (-1.1392, 5.472) (-1.1442, 5.4776) (-1.1493, 5.4833) (-1.1545, 5.489) (-1.1596, 5.4946) (-1.1648, 5.5003) (-1.1701, 5.506) (-1.1753, 5.5117) (-1.1806, 5.5174) (-1.1859, 5.5231) (-1.1913, 5.5288) (-1.1967, 5.5345) (-1.2021, 5.5402) (-1.2076, 5.5459) (-1.2131, 5.5517) (-1.2186, 5.5574) (-1.2242, 5.5631) (-1.2298, 5.5688) (-1.2354, 5.5746) (-1.2411, 5.5803) (-1.2468, 5.5861) (-1.2525, 5.5918) (-1.2583, 5.5976) (-1.264, 5.6033) (-1.2699, 5.6091) (-1.2757, 5.6148) (-1.2816, 5.6206) (-1.2876, 5.6264) (-1.2935, 5.6321) (-1.2995, 5.6379) (-1.3055, 5.6437) (-1.3116, 5.6494) (-1.3177, 5.6552) (-1.3238, 5.661) (-1.33, 5.6667) (-1.3362, 5.6725) (-1.3424, 5.6783) (-1.3487, 5.6841) (-1.355, 5.6898) (-1.3613, 5.6956) (-1.3676, 5.7014) (-1.374, 5.7072) (-1.3805, 5.7129) (-1.3869, 5.7187) (-1.3934, 5.7245) (-1.3999, 5.7302) (-1.4065, 5.736) (-1.4131, 5.7418) (-1.4197, 5.7475) (-1.4264, 5.7533) (-1.433, 5.7591) (-1.4398, 5.7648) (-1.4465, 5.7706) (-1.4533, 5.7764) (-1.4601, 5.7821) (-1.467, 5.7879) (-1.4739, 5.7936) (-1.4808, 5.7994) (-1.4863, 5.8039) (-1.4905, 5.8074) (-1.4933, 5.8097) (-1.4947, 5.8108) knots 0 0 0 0 0 0 0.00416667 0.00833333 0.0125 0.01666667 0.02083333 0.025 0.02916667 0.03333333 0.0375 0.04166667 0.04583333 0.05 0.05416667 0.05833333 0.0625 0.06666667 0.07083333 0.075 0.07916667 0.08333333 0.0875 0.09166667 0.09583333 0.1 0.10416667 0.10833333 0.1125 0.11666667 0.12083333 0.125 0.12916667 0.13333333 0.1375 0.14166667 0.14583333 0.15 0.15416667 0.15833333 0.1625 0.16666667 0.17083333 0.175 0.17916667 0.18333333 0.1875 0.19166667 0.19583333 0.2 0.20416667 0.20833333 0.2125 0.21666667 0.22083333 0.225 0.22916667 0.23333333 0.2375 0.24166667 0.24583333 0.25 0.25416667 0.25833333 0.2625 0.26666667 0.27083333 0.275 0.27916667 0.28333333 0.2875 0.29166667 0.29583333 0.3 0.30416667 0.30833333 0.3125 0.31666667 0.32083333 0.325 0.32916667 0.33333333 0.3375 0.34166667 0.34583333 0.35 0.35416667 0.35833333 0.3625 0.36666667 0.37083333 0.375 0.37916667 0.38333333 0.3875 0.39166667 0.39583333 0.4 0.40416667 0.40833333 0.4125 0.41666667 0.42083333 0.425 0.42916667 0.43333333 0.4375 0.44166667 0.44583333 0.45 0.45416667 0.45833333 0.4625 0.46666667 0.47083333 0.475 0.47916667 0.48333333 0.4875 0.49166667 0.49583333 0.5 0.50416667 0.50833333 0.5125 0.51666667 0.52083333 0.525 0.52916667 0.53333333 0.5375 0.54166667 0.54583333 0.55 0.55416667 0.55833333 0.5625 0.56666667 0.57083333 0.575 0.57916667 0.58333333 0.5875 0.59166667 0.59583333 0.6 0.60416667 0.60833333 0.6125 0.61666667 0.62083333 0.625 0.62916667 0.63333333 0.6375 0.64166667 0.64583333 0.65 0.65416667 0.65833333 0.6625 0.66666667 0.67083333 0.675 0.67916667 0.68333333 0.6875 0.69166667 0.69583333 0.7 0.70416667 0.70833333 0.7125 0.71666667 0.72083333 0.725 0.72916667 0.73333333 0.7375 0.74166667 0.74583333 0.75 0.75416667 0.75833333 0.7625 0.76666667 0.77083333 0.775 0.77916667 0.78333333 0.7875 0.79166667 0.79583333 0.8 0.80416667 0.80833333 0.8125 0.81666667 0.82083333 0.825 0.82916667 0.83333333 0.8375 0.84166667 0.84583333 0.85 0.85416667 0.85833333 0.8625 0.86666667 0.87083333 0.875 0.87916667 0.88333333 0.8875 0.89166667 0.89583333 0.9 0.90416667 0.90833333 0.9125 0.91666667 0.92083333 0.925 0.92916667 0.93333333 0.9375 0.94166667 0.94583333 0.95 0.95416667 0.95833333 0.9625 0.96666667 0.97083333 0.975 0.97916667 0.98333333 0.9875 0.99166667 0.99583333 1 1 1 1 1 1
  arc A17 (-1.4947, 5.8108) -> (-2.2063, 5.5796) centre (0, 0) ccw
  spline S17 degree 5 poles (-2.2063, 5.5796) (-2.2067, 5.5779) (-2.2076, 5.5744) (-2.209, 5.5691) (-2.2108, 5.5622) (-2.213, 5.5534) (-2.2152, 5.5447) (-2.2174, 5.5361) (-2.2195, 5.5274) (-2.2216, 5.5188) (-2.2237, 5.5101) (-2.2257, 5.5015) (-2.2278, 5.4929) (-2.2298, 5.4843) (-2.2317, 5.4758) (-2.2337, 5.4672) (-2.2356, 5.4587) (-2.2375, 5.4502) (-2.2393, 5.4417) (-2.2412, 5.4333) (-2.243, 5.4248) (-2.2447, 5.4164) (-2.2465, 5.408) (-2.2482, 5.3996) (-2.2499, 5.3912) (-2.2516, 5.3829) (-2.2532, 5.3746) (-2.2548, 5.3662) (-2.2564, 5.358) (-2.258, 5.3497) (-2.2595, 5.3414) (-2.2611, 5.3332) (-2.2625, 5.325) (-2.264, 5.3168) (-2.2654, 5.3086) (-2.2668, 5.3005) (-2.2682, 5.2924) (-2.2696, 5.2843) (-2.2709, 5.2762) (-2.2722, 5.2681) (-2.2735, 5.2601) (-2.2748, 5.2521) (-2.276, 5.2441) (-2.2772, 5.2361) (-2.2784, 5.2281) (-2.2795, 5.2202) (-2.2807, 5.2123) (-2.2818, 5.2044) (-2.2829, 5.1966) (-2.2839, 5.1887) (-2.2849, 5.1809) (-2.286, 5.1731) (-2.2869, 5.1653) (-2.2879, 5.1576) (-2.2888, 5.1499) (-2.2897, 5.1422) (-2.2906, 5.1345) (-2.2915, 5.1269) (-2.2923, 5.1192) (-2.2932, 5.1116) (-2.294, 5.1041) (-2.2947, 5.0965) (-2.2955, 5.089) (-2.2962, 5.0815) (-2.2969, 5.074) (-2.2976, 5.0666) (-2.2982, 5.0591) (-2.2989, 5.0517) (-2.2995, 5.0444) (-2.3001, 5.037) (-2.3006, 5.0297) (-2.3012, 5.0224) (-2.3017, 5.0151) (-2.3022, 5.0079) (-2.3027, 5.0007) (-2.3031, 4.9935) (-2.3036, 4.9863) (-2.304, 4.9792) (-2.3044, 4.9721) (-2.3048, 4.965) (-2.3051, 4.9579) (-2.3054, 4.9509) (-2.3057, 4.9439) (-2.306, 4.937) (-2.3063, 4.93) (-2.3066, 4.9231) (-2.3068, 4.9162) (-2.307, 4.9094) (-2.3072, 4.9025) (-2.3073, 4.8958) (-2.3075, 4.889) (-2.3076, 4.8822) (-2.3077, 4.8755) (-2.3078, 4.8689) (-2.3079, 4.8622) (-2.3079, 4.8556) (-2.308, 4.849) (-2.308, 4.8424) (-2.308, 4.8359) (-2.308, 4.8294) (-2.3079, 4.823) (-2.3079, 4.8165) (-2.3078, 4.8101) (-2.3077, 4.8037) (-2.3076, 4.7974) (-2.3074, 4.7911) (-2.3073, 4.7848) (-2.3071, 4.7786) (-2.307, 4.7724) (-2.3068, 4.7662) (-2.3065, 4.76) (-2.3063, 4.7539) (-2.3061, 4.7478) (-2.3058, 4.7418) (-2.3055, 4.7357) (-2.3052, 4.7298) (-2.3049, 4.7238) (-2.3046, 4.7179) (-2.3042, 4.712) (-2.3039, 4.7062) (-2.3035, 4.7003) (-2.3031, 4.6945) (-2.3027, 4.6888) (-2.3023, 4.6831) (-2.3019, 4.6774) (-2.3014, 4.6718) (-2.301, 4.6661) (-2.3005, 4.6606) (-2.3, 4.655) (-2.2995, 4.6495) (-2.299, 4.6441) (-2.2985, 4.6386) (-2.2979, 4.6332) (-2.2974, 4.6279) (-2.2968, 4.6225) (-2.2963, 4.6173) (-2.2957, 4.612) (-2.2951, 4.6068) (-2.2945, 4.6016) (-2.2938, 4.5965) (-2.2932, 4.5914) (-2.2926, 4.5863) (-2.2919, 4.5813) (-2.2913, 4.5763) (-2.2906, 4.5713) (-2.2899, 4.5664) (-2.2892, 4.5616) (-2.2885, 4.5567) (-2.2878, 4.5519) (-2.2871, 4.5472) (-2.2863, 4.5424) (-2.2856, 4.5378) (-2.2849, 4.5331) (-2.2841, 4.5285) (-2.2833, 4.524) (-2.2826, 4.5194) (-2.2818, 4.515) (-2.281, 4.5105) (-2.2802, 4.5061) (-2.2794, 4.5018) (-2.2786, 4.4974) (-2.2778, 4.4932) (-2.277, 4.4889) (-2.2762, 4.4847) (-2.2753, 4.4806) (-2.2745, 4.4765) (-2.2737, 4.4724) (-2.2728, 4.4684) (-2.272, 4.4644) (-2.2711, 4.4604) (-2.2703, 4.4565) (-2.2694, 4.4527) (-2.2686, 4.4489) (-2.2677, 4.4451) (-2.2668, 4.4414) (-2.266, 4.4377) (-2.2651, 4.4341) (-2.2642, 4.4305) (-2.2634, 4.4269) (-2.2625, 4.4234) (-2.2616, 4.4199) (-2.2608, 4.4165) (-2.2599, 4.4132) (-2.259, 4.4098) (-2.2581, 4.4066) (-2.2573, 4.4033) (-2.2564, 4.4001) (-2.2555, 4.397) (-2.2547, 4.3939) (-2.2538, 4.3908) (-2.2529, 4.3878) (-2.2521, 4.3849) (-2.2512, 4.382) (-2.2504, 4.3791) (-2.2495, 4.3763) (-2.2487, 4.3735) (-2.2478, 4.3708) (-2.247, 4.3681) (-2.2462, 4.3655) (-2.2453, 4.3629) (-2.2445, 4.3604) (-2.2437, 4.3579) (-2.2429, 4.3555) (-2.2421, 4.3531) (-2.2413, 4.3508) (-2.2405, 4.3485) (-2.2398, 4.3463) (-2.239, 4.3441) (-2.2383, 4.342) (-2.2375, 4.3399) (-2.2368, 4.3379) (-2.2361, 4.3359) (-2.2354, 4.334) (-2.2347, 4.3321) (-2.234, 4.3303) (-2.2333, 4.3285) (-2.2326, 4.3268) (-2.232, 4.3251) (-2.2314, 4.3235) (-2.2307, 4.322) (-2.2301, 4.3205) (-2.2296, 4.319) (-2.229, 4.3176) (-2.2284, 4.3163) (-2.2279, 4.315) (-2.2274, 4.3138) (-2.2269, 4.3126) (-2.2264, 4.3115) (-2.2259, 4.3104) (-2.2255, 4.3094) (-2.2251, 4.3084) (-2.2247, 4.3075) (-2.2243, 4.3067) (-2.2239, 4.3059) (-2.2236, 4.3051) (-2.2233, 4.3045) (-2.223, 4.3038) (-2.2227, 4.3033) (-2.2225, 4.3028) (-2.2223, 4.3023) (-2.2221, 4.3019) (-2.2219, 4.3017) (-2.2218, 4.3015) (-2.2218, 4.3014) (-2.2218, 4.3014) knots -1 -1 -1 -1 -1 -1 -0.99583333 -0.99166667 -0.9875 -0.98333333 -0.97916667 -0.975 -0.97083333 -0.96666667 -0.9625 -0.95833333 -0.95416667 -0.95 -0.94583333 -0.94166667 -0.9375 -0.93333333 -0.92916667 -0.925 -0.92083333 -0.91666667 -0.9125 -0.90833333 -0.90416667 -0.9 -0.89583333 -0.89166667 -0.8875 -0.88333333 -0.87916667 -0.875 -0.87083333 -0.86666667 -0.8625 -0.85833333 -0.85416667 -0.85 -0.84583333 -0.84166667 -0.8375 -0.83333333 -0.82916667 -0.825 -0.82083333 -0.81666667 -0.8125 -0.80833333 -0.80416667 -0.8 -0.79583333 -0.79166667 -0.7875 -0.78333333 -0.77916667 -0.775 -0.77083333 -0.76666667 -0.7625 -0.75833333 -0.75416667 -0.75 -0.74583333 -0.74166667 -0.7375 -0.73333333 -0.72916667 -0.725 -0.72083333 -0.71666667 -0.7125 -0.70833333 -0.70416667 -0.7 -0.69583333 -0.69166667 -0.6875 -0.68333333 -0.67916667 -0.675 -0.67083333 -0.66666667 -0.6625 -0.65833333 -0.65416667 -0.65 -0.64583333 -0.64166667 -0.6375 -0.63333333 -0.62916667 -0.625 -0.62083333 -0.61666667 -0.6125 -0.60833333 -0.60416667 -0.6 -0.59583333 -0.59166667 -0.5875 -0.58333333 -0.57916667 -0.575 -0.57083333 -0.56666667 -0.5625 -0.55833333 -0.55416667 -0.55 -0.54583333 -0.54166667 -0.5375 -0.53333333 -0.52916667 -0.525 -0.52083333 -0.51666667 -0.5125 -0.50833333 -0.50416667 -0.5 -0.49583333 -0.49166667 -0.4875 -0.48333333 -0.47916667 -0.475 -0.47083333 -0.46666667 -0.4625 -0.45833333 -0.45416667 -0.45 -0.44583333 -0.44166667 -0.4375 -0.43333333 -0.42916667 -0.425 -0.42083333 -0.41666667 -0.4125 -0.40833333 -0.40416667 -0.4 -0.39583333 -0.39166667 -0.3875 -0.38333333 -0.37916667 -0.375 -0.37083333 -0.36666667 -0.3625 -0.35833333 -0.35416667 -0.35 -0.34583333 -0.34166667 -0.3375 -0.33333333 -0.32916667 -0.325 -0.32083333 -0.31666667 -0.3125 -0.30833333 -0.30416667 -0.3 -0.29583333 -0.29166667 -0.2875 -0.28333333 -0.27916667 -0.275 -0.27083333 -0.26666667 -0.2625 -0.25833333 -0.25416667 -0.25 -0.24583333 -0.24166667 -0.2375 -0.23333333 -0.22916667 -0.225 -0.22083333 -0.21666667 -0.2125 -0.20833333 -0.20416667 -0.2 -0.19583333 -0.19166667 -0.1875 -0.18333333 -0.17916667 -0.175 -0.17083333 -0.16666667 -0.1625 -0.15833333 -0.15416667 -0.15 -0.14583333 -0.14166667 -0.1375 -0.13333333 -0.12916667 -0.125 -0.12083333 -0.11666667 -0.1125 -0.10833333 -0.10416667 -0.1 -0.09583333 -0.09166667 -0.0875 -0.08333333 -0.07916667 -0.075 -0.07083333 -0.06666667 -0.0625 -0.05833333 -0.05416667 -0.05 -0.04583333 -0.04166667 -0.0375 -0.03333333 -0.02916667 -0.025 -0.02083333 -0.01666667 -0.0125 -0.00833333 -0.00416667 0 0 0 0 0 0
  line L34 (-2.2218, 4.3014) -> (-2.2215, 4.3009)
  line L35 (-2.2215, 4.3009) -> (-1.721, 3.3318)
  arc A18 (-1.721, 3.3318) -> (-2.6369, 2.6663) centre (0, 0) ccw
  line L36 (-2.6369, 2.6663) -> (-3.4039, 3.4418)
  line L37 (-3.4039, 3.4418) -> (-3.4043, 3.4422)